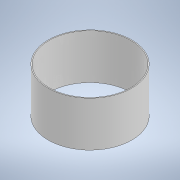
# Autodesk Inventor part: 18650
Saved by Autodesk Inventor 2020.1 (Build 241239000, 239)
## iProperties
Created: 2023-01-08
Part Number: 18650
Material: Типовые
Document SubType Name: Modeling
Designer: KirikDK
Density: 1 g/cm^3
Appearance: По умолчанию
Author: KirikDK
Autodesk Inventor part; units mm, degrees
ref_plane "YZ Plane" through (0, 0, 0) normal (1, 0, 0) x (0, 1, 0)
ref_plane "XZ Plane" through (0, 0, 0) normal (0, 1, 0) x (-1, 0, 0)
ref_plane "XY Plane" through (0, 0, 0) normal (0, 0, 1) x (1, 0, 0)
sketch "Эскиз1" plane through (0, 0, 0) normal (0, 1, 0) x (-1, 0, 0)
  circle A0 centre (0, 0) radius 9.1
  line L0 (0, -10.7442) -> (-9.3048, -5.3721)
  line L1 (-9.3048, -5.3721) -> (-9.3048, 5.3721)
  line L2 (-9.3048, 5.3721) -> (0, 10.7442)
  line L3 (0, 10.7442) -> (9.3048, 5.3721)
  line L4 (9.3048, 5.3721) -> (9.3048, -5.3721)
  line L5 (9.3048, -5.3721) -> (0, -10.7442)
  circle A1 centre (0, 0) radius 9.3048
  dimension "d0" = 18.2
  constraints: 12 end point, 3 coincident, 2 centre point, 1 tangent, 13 other
  measures "d0" diameter of A0
extrude "Выдавливание1" add sketch "Эскиз1" along normal blind 10 contours A1
